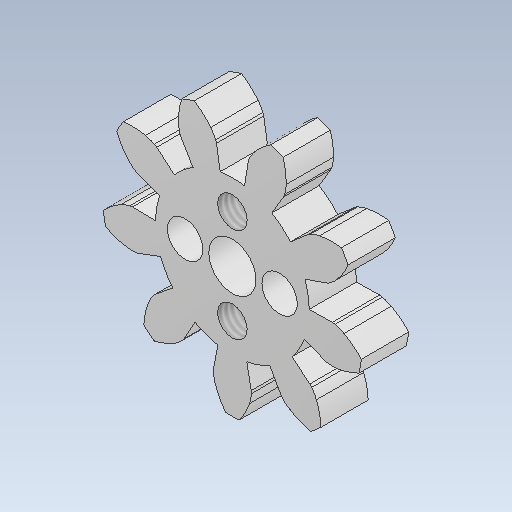
# Autodesk Inventor part: ｍ2歯数9ギアd3.99
Saved by Autodesk Inventor 2020.2 (Build 242310000, 310)
## iProperties
Created: 2020-03-11
Part Number: ｍ2歯数9ギアd3.99
Material: アルミニウム 2014-T4
Document SubType Name: Modeling
Designer: aoyam
Density: 2.8 g/cm^3
Appearance: サテン
Mass: 2.2827 g
Surface Area: 10.6305 cm^2
Volume: 0.815251 cm^3
Author: aoyam
Autodesk Inventor part; units mm, degrees
ref_plane "YZ Plane" through (0, 0, 0) normal (1, 0, 0) x (0, 1, 0)
ref_plane "XZ Plane" through (0, 0, 0) normal (0, 1, 0) x (-1, 0, 0)
ref_plane "XY Plane" through (0, 0, 0) normal (0, 0, 1) x (1, 0, 0)
sketch "スケッチ1" plane through (0, 0, 0) normal (0, 0, 1) x (1, 0, 0)
  arc A0 (8.759, 12.6536) -> (8.6861, 12.4312) centre (9.7767, 12.197) ccw
  arc A1 (9.1794, 13.3512) -> (8.759, 12.6536) centre (11.6212, 11.4041) ccw
  arc A2 (10.5668, 14.5981) -> (9.1794, 13.3512) centre (13.5776, 9.8526) ccw
  arc A3 (5.9975, 12.4312) -> (5.9246, 12.6536) centre (4.9069, 12.197) ccw
  arc A4 (5.9246, 12.6536) -> (5.5042, 13.3512) centre (3.0623, 11.4041) ccw
  arc A5 (5.5042, 13.3512) -> (4.1168, 14.5981) centre (1.106, 9.8526) ccw
  arc A6 (8.375, 10.4988) -> (6.3086, 10.4988) centre (7.3418, 4.0815) ccw
  arc A7 (4.1168, 14.5981) -> (3.0523, 14.2107) centre (7.3418, 4.0815) ccw
  line L0 (8.375, 10.4988) -> (8.6861, 12.4312)
  line L1 (6.3086, 10.4988) -> (5.9975, 12.4312)
  line L2 (2.4253, 8.3333) -> (0.9449, 9.6136)
  arc A8 (0.9449, 9.6136) -> (0.7461, 9.7372) centre (0.26, 8.7332) ccw
  arc A9 (0.7461, 9.7372) -> (-0.0244, 10.0013) centre (-0.6433, 6.9401) ccw
  arc A10 (-0.0244, 10.0013) -> (-1.8887, 10.0647) centre (-1.1447, 4.4942) ccw
  arc A11 (-1.8887, 10.0647) -> (-2.455, 9.0837) centre (7.3418, 4.0815) ccw
  arc A12 (2.9173, 11.5591) -> (3.0045, 11.3418) centre (3.9905, 11.8635) ccw
  arc A13 (4.0083, 9.6616) -> (2.4253, 8.3333) centre (7.3418, 4.0815) ccw
  line L3 (4.0083, 9.6616) -> (3.0045, 11.3418)
  arc A14 (2.791, 12.3637) -> (2.9173, 11.5591) centre (5.9132, 12.4417) ccw
  arc A15 (3.0523, 14.2107) -> (2.791, 12.3637) centre (8.409, 12.5107) ccw
  line L4 (0.8425, 4.1783) -> (-1.1145, 4.2075)
  arc A16 (-1.1145, 4.2075) -> (-1.3462, 4.1744) centre (-1.0733, 3.0928) ccw
  arc A17 (-1.3462, 4.1744) -> (-2.1062, 3.8815) centre (-0.6127, 1.1386) ccw
  arc A18 (-2.1062, 3.8815) -> (-3.5751, 2.7316) centre (0.5755, -1.0574) ccw
  arc A19 (-3.5751, 2.7316) -> (-3.3784, 1.6161) centre (7.3418, 4.0815) ccw
  arc A20 (-0.8541, 6.9657) -> (-0.6476, 6.8552) centre (-0.2276, 7.8886) ccw
  arc A21 (1.2013, 6.2133) -> (0.8425, 4.1783) centre (7.3418, 4.0815) ccw
  line L5 (1.2013, 6.2133) -> (-0.6476, 6.8552)
  arc A22 (-1.468, 7.5008) -> (-0.8541, 6.9657) centre (0.8736, 9.5675) ccw
  arc A23 (-2.455, 9.0837) -> (-1.468, 7.5008) centre (2.7411, 11.2246) ccw
  line L6 (2.3008, -0.022) -> (0.7829, -1.2576)
  arc A24 (0.7829, -1.2576) -> (0.6267, -1.4319) centre (1.531, -2.085) ccw
  arc A25 (0.6267, -1.4319) -> (0.2328, -2.1448) centre (3.14, -3.286) ccw
  arc A26 (0.2328, -2.1448) -> (-0.1534, -3.9698) centre (5.4617, -4.2045) ccw
  arc A27 (-0.1534, -3.9698) -> (0.7144, -4.6979) centre (7.3418, 4.0815) ccw
  arc A28 (-0.7905, 1.0227) -> (-0.5614, 1.0708) centre (-0.9039, 2.1324) ccw
  arc A29 (1.2676, 1.7675) -> (2.3008, -0.022) centre (7.3418, 4.0815) ccw
  line L7 (1.2676, 1.7675) -> (-0.5614, 1.0708)
  arc A30 (-1.6048, 1.038) -> (-0.7905, 1.0227) centre (-1.1395, 4.1263) ccw
  arc A31 (-3.3784, 1.6161) -> (-1.6048, 1.038) centre (-0.7741, 6.5962) ccw
  line L8 (6.1178, -2.3023) -> (5.7492, -4.2245)
  arc A32 (5.7492, -4.2245) -> (5.7416, -4.4585) centre (6.8542, -4.3774) ccw
  arc A33 (5.7416, -4.4585) -> (5.8981, -5.2577) centre (8.8587, -4.2632) ccw
  arc A34 (5.8981, -5.2577) -> (6.7754, -6.9039) centre (11.2276, -3.4744) ccw
  arc A35 (6.7754, -6.9039) -> (7.9082, -6.9039) centre (7.3418, 4.0815) ccw
  arc A36 (3.0782, -3.489) -> (3.2228, -3.3049) centre (2.278, -2.7119) ccw
  arc A37 (4.176, -1.5955) -> (6.1178, -2.3023) centre (7.3418, 4.0815) ccw
  line L9 (4.176, -1.5955) -> (3.2228, -3.3049)
  arc A38 (2.4446, -4.0008) -> (3.0782, -3.489) centre (0.8159, -1.3359) ccw
  arc A39 (0.7144, -4.6979) -> (2.4446, -4.0008) centre (-0.4918, 0.7911) ccw
  line L10 (10.5075, -1.5955) -> (11.4608, -3.3049)
  arc A40 (11.4608, -3.3049) -> (11.6054, -3.489) centre (12.4055, -2.7119) ccw
  arc A41 (11.6054, -3.489) -> (12.239, -4.0008) centre (13.8676, -1.3359) ccw
  arc A42 (12.239, -4.0008) -> (13.9692, -4.6979) centre (15.1754, 0.7911) ccw
  arc A43 (13.9692, -4.6979) -> (14.8369, -3.9698) centre (7.3418, 4.0815) ccw
  arc A44 (8.9419, -4.4585) -> (8.9343, -4.2245) centre (7.8294, -4.3774) ccw
  arc A45 (8.5658, -2.3023) -> (10.5075, -1.5955) centre (7.3418, 4.0815) ccw
  line L11 (8.5658, -2.3023) -> (8.9343, -4.2245)
  arc A46 (8.7855, -5.2577) -> (8.9419, -4.4585) centre (5.8249, -4.2632) ccw
  arc A47 (7.9082, -6.9039) -> (8.7855, -5.2577) centre (3.4559, -3.4744) ccw
  line L12 (13.416, 1.7675) -> (15.245, 1.0708)
  arc A48 (15.245, 1.0708) -> (15.4741, 1.0227) centre (15.5875, 2.1324) ccw
  arc A49 (15.4741, 1.0227) -> (16.2884, 1.038) centre (15.8231, 4.1263) ccw
  arc A50 (16.2884, 1.038) -> (18.062, 1.6161) centre (15.4577, 6.5962) ccw
  arc A51 (18.062, 1.6161) -> (18.2587, 2.7316) centre (7.3418, 4.0815) ccw
  arc A52 (14.0569, -1.4319) -> (13.9007, -1.2576) centre (13.1526, -2.085) ccw
  arc A53 (12.3828, -0.022) -> (13.416, 1.7675) centre (7.3418, 4.0815) ccw
  line L13 (12.3828, -0.022) -> (13.9007, -1.2576)
  arc A54 (14.4508, -2.1448) -> (14.0569, -1.4319) centre (11.5436, -3.286) ccw
  arc A55 (14.8369, -3.9698) -> (14.4508, -2.1448) centre (9.2219, -4.2045) ccw
  line L14 (13.4822, 6.2133) -> (15.3312, 6.8552)
  arc A56 (15.3312, 6.8552) -> (15.5376, 6.9657) centre (14.9112, 7.8886) ccw
  arc A57 (15.5376, 6.9657) -> (16.1516, 7.5008) centre (13.81, 9.5675) ccw
  arc A58 (16.1516, 7.5008) -> (17.1386, 9.0837) centre (11.9425, 11.2246) ccw
  arc A59 (17.1386, 9.0837) -> (16.5722, 10.0647) centre (7.3418, 4.0815) ccw
  arc A60 (16.0298, 4.1744) -> (15.7981, 4.2075) centre (15.7569, 3.0928) ccw
  arc A61 (13.8411, 4.1783) -> (13.4822, 6.2133) centre (7.3418, 4.0815) ccw
  line L15 (13.8411, 4.1783) -> (15.7981, 4.2075)
  arc A62 (16.7898, 3.8815) -> (16.0298, 4.1744) centre (15.2963, 1.1386) ccw
  arc A63 (18.2587, 2.7316) -> (16.7898, 3.8815) centre (14.1081, -1.0574) ccw
  line L16 (10.6753, 9.6616) -> (11.6791, 11.3418)
  arc A64 (11.6791, 11.3418) -> (11.7663, 11.5591) centre (10.6931, 11.8635) ccw
  arc A65 (11.7663, 11.5591) -> (11.8926, 12.3637) centre (8.7704, 12.4417) ccw
  arc A66 (11.8926, 12.3637) -> (11.6312, 14.2107) centre (6.2746, 12.5107) ccw
  arc A67 (11.6312, 14.2107) -> (10.5668, 14.5981) centre (7.3418, 4.0815) ccw
  arc A68 (13.9375, 9.7372) -> (13.7387, 9.6136) centre (14.4236, 8.7332) ccw
  arc A69 (12.2583, 8.3333) -> (10.6753, 9.6616) centre (7.3418, 4.0815) ccw
  line L17 (12.2583, 8.3333) -> (13.7387, 9.6136)
  arc A70 (14.7079, 10.0013) -> (13.9375, 9.7372) centre (15.3269, 6.9401) ccw
  arc A71 (16.5722, 10.0647) -> (14.7079, 10.0013) centre (15.8283, 4.4942) ccw
  circle A72 centre (7.3418, 4.0815) radius 1.995
  point P0 (0, 0)
  point P1 (6.3086, 10.4988)
  point P2 (5.9975, 12.4312)
  point P3 (5.9246, 12.6536)
  point P4 (5.5094, 13.3447)
  point P5 (4.1168, 14.5981)
  point P6 (3.0523, 14.2107)
  point P7 (2.7912, 12.3553)
  point P8 (2.9173, 11.5591)
  point P9 (3.0045, 11.3418)
  point P10 (4.0083, 9.6616)
  point P11 (2.4253, 8.3333)
  point P12 (0.9449, 9.6136)
  point P13 (0.7461, 9.7372)
  point P14 (-0.0162, 9.9996)
  point P15 (-1.8887, 10.0647)
  point P16 (-2.455, 9.0837)
  point P17 (-1.4625, 7.4946)
  point P18 (-0.8541, 6.9657)
  point P19 (-0.6476, 6.8552)
  point P20 (1.2013, 6.2133)
  point P21 (0.8425, 4.1783)
  point P22 (-1.1145, 4.2075)
  point P23 (-1.3462, 4.1744)
  point P24 (-2.0989, 3.8854)
  point P25 (-3.5751, 2.7316)
  point P26 (-3.3784, 1.6161)
  point P27 (-1.5966, 1.0368)
  point P28 (-0.7905, 1.0227)
  point P29 (-0.5614, 1.0708)
  point P30 (2.3008, -0.022)
  point P31 (0.7829, -1.2576)
  point P32 (0.6267, -1.4319)
  point P33 (0.2358, -2.137)
  point P34 (-0.1534, -3.9698)
  point P35 (0.7144, -4.6979)
  point P36 (2.4517, -3.9964)
  point P37 (3.0782, -3.489)
  point P38 (3.2228, -3.3049)
  point P39 (6.1178, -2.3023)
  point P40 (5.7492, -4.2245)
  point P41 (5.7416, -4.4585)
  point P42 (5.8955, -5.2498)
  point P43 (6.7754, -6.9039)
  point P44 (7.9082, -6.9039)
  point P45 (8.7881, -5.2498)
  point P46 (8.9419, -4.4585)
  point P47 (8.9343, -4.2245)
  point P48 (8.5658, -2.3023)
  point P49 (11.6054, -3.489)
  point P50 (12.2319, -3.9964)
  point P51 (13.9692, -4.6979)
  point P52 (14.8369, -3.9698)
  point P53 (14.4478, -2.137)
  point P54 (14.0569, -1.4319)
  point P55 (13.9007, -1.2576)
  point P56 (12.3828, -0.022)
  point P57 (13.416, 1.7675)
  point P58 (15.4741, 1.0227)
  point P59 (16.2802, 1.0368)
  point P60 (18.062, 1.6161)
  point P61 (18.2587, 2.7316)
  point P62 (16.7825, 3.8854)
  point P63 (16.0298, 4.1744)
  point P64 (15.7981, 4.2075)
  point P65 (13.8411, 4.1783)
  point P66 (15.5376, 6.9657)
  point P67 (16.1461, 7.4946)
  point P68 (17.1386, 9.0837)
  point P69 (16.5722, 10.0647)
  point P70 (14.6998, 9.9996)
  point P71 (13.9375, 9.7372)
  point P72 (11.7663, 11.5591)
  point P73 (11.8924, 12.3553)
  point P74 (10.5668, 14.5981)
  point P75 (9.1742, 13.3447)
  point P76 (8.759, 12.6536)
  dimension "d2" = 360
  dimension "d4" = 3.99
  constraints: 144 point on circle, 73 centre point, 36 end point, 3 coincident, 341 other
  measures "d4" diameter of A72
extrude "押し出し1" add sketch "スケッチ1" along normal blind 4
sketch "スケッチ4" plane through (0, 0, 4) normal (0, 0, 1) x (1, 0, 0)
  arc A0 (5.9975, 12.4312) -> (5.9246, 12.6536) centre (4.9069, 12.197) ccw projected
  arc A1 (5.9246, 12.6536) -> (5.5094, 13.3447) centre (3.0623, 11.4041) ccw projected
  arc A2 (5.5094, 13.3447) -> (4.1168, 14.5981) centre (1.106, 9.8526) ccw projected
  arc A3 (4.1168, 14.5981) -> (3.0523, 14.2107) centre (7.3418, 4.0815) ccw projected
  arc A4 (3.0523, 14.2107) -> (2.791, 12.3637) centre (8.409, 12.5107) ccw projected
  arc A5 (2.791, 12.3637) -> (2.9173, 11.5591) centre (5.9132, 12.4417) ccw projected
  arc A6 (2.9173, 11.5591) -> (3.0045, 11.3418) centre (3.9905, 11.8635) ccw projected
  line L0 (3.0045, 11.3418) -> (4.0083, 9.6616) projected
  arc A7 (4.0083, 9.6616) -> (2.4253, 8.3333) centre (7.3418, 4.0815) ccw projected
  line L1 (2.4253, 8.3333) -> (0.9449, 9.6136) projected
  arc A8 (0.9449, 9.6136) -> (0.7461, 9.7372) centre (0.26, 8.7332) ccw projected
  arc A9 (0.7461, 9.7372) -> (-0.0162, 9.9996) centre (-0.6433, 6.9401) ccw projected
  arc A10 (-0.0162, 9.9996) -> (-1.8887, 10.0647) centre (-1.1447, 4.4942) ccw projected
  arc A11 (-1.8887, 10.0647) -> (-2.455, 9.0837) centre (7.3418, 4.0815) ccw projected
  arc A12 (-2.455, 9.0837) -> (-1.468, 7.5008) centre (2.7411, 11.2246) ccw projected
  arc A13 (-1.468, 7.5008) -> (-0.8541, 6.9657) centre (0.8736, 9.5675) ccw projected
  arc A14 (-0.8541, 6.9657) -> (-0.6476, 6.8552) centre (-0.2276, 7.8886) ccw projected
  line L2 (-0.6476, 6.8552) -> (1.2013, 6.2133) projected
  arc A15 (1.2013, 6.2133) -> (0.8425, 4.1783) centre (7.3418, 4.0815) ccw projected
  line L3 (0.8425, 4.1783) -> (-1.1145, 4.2075) projected
  arc A16 (-1.1145, 4.2075) -> (-1.3462, 4.1744) centre (-1.0733, 3.0928) ccw projected
  arc A17 (-1.3462, 4.1744) -> (-2.0989, 3.8854) centre (-0.6127, 1.1386) ccw projected
  arc A18 (-2.0989, 3.8854) -> (-3.5751, 2.7316) centre (0.5755, -1.0574) ccw projected
  arc A19 (-3.5751, 2.7316) -> (-3.3784, 1.6161) centre (7.3418, 4.0815) ccw projected
  arc A20 (-3.3784, 1.6161) -> (-1.6048, 1.038) centre (-0.7741, 6.5962) ccw projected
  arc A21 (-1.6048, 1.038) -> (-0.7905, 1.0227) centre (-1.1395, 4.1263) ccw projected
  arc A22 (-0.7905, 1.0227) -> (-0.5614, 1.0708) centre (-0.9039, 2.1324) ccw projected
  line L4 (-0.5614, 1.0708) -> (1.2676, 1.7675) projected
  arc A23 (1.2676, 1.7675) -> (2.3008, -0.022) centre (7.3418, 4.0815) ccw projected
  line L5 (2.3008, -0.022) -> (0.7829, -1.2576) projected
  arc A24 (0.7829, -1.2576) -> (0.6267, -1.4319) centre (1.531, -2.085) ccw projected
  arc A25 (0.6267, -1.4319) -> (0.2358, -2.137) centre (3.14, -3.286) ccw projected
  arc A26 (0.2358, -2.137) -> (-0.1534, -3.9698) centre (5.4617, -4.2045) ccw projected
  arc A27 (-0.1534, -3.9698) -> (0.7144, -4.6979) centre (7.3418, 4.0815) ccw projected
  arc A28 (0.7144, -4.6979) -> (2.4446, -4.0008) centre (-0.4918, 0.7911) ccw projected
  arc A29 (2.4446, -4.0008) -> (3.0782, -3.489) centre (0.8159, -1.3359) ccw projected
  arc A30 (3.0782, -3.489) -> (3.2228, -3.3049) centre (2.278, -2.7119) ccw projected
  line L6 (3.2228, -3.3049) -> (4.176, -1.5955) projected
  arc A31 (4.176, -1.5955) -> (6.1178, -2.3023) centre (7.3418, 4.0815) ccw projected
  line L7 (6.1178, -2.3023) -> (5.7492, -4.2245) projected
  arc A32 (5.7492, -4.2245) -> (5.7416, -4.4585) centre (6.8542, -4.3774) ccw projected
  arc A33 (5.7416, -4.4585) -> (5.8955, -5.2498) centre (8.8587, -4.2632) ccw projected
  arc A34 (5.8955, -5.2498) -> (6.7754, -6.9039) centre (11.2276, -3.4744) ccw projected
  arc A35 (6.7754, -6.9039) -> (7.9082, -6.9039) centre (7.3418, 4.0815) ccw projected
  arc A36 (7.9082, -6.9039) -> (8.7855, -5.2577) centre (3.4559, -3.4744) ccw projected
  arc A37 (8.7855, -5.2577) -> (8.9419, -4.4585) centre (5.8249, -4.2632) ccw projected
  arc A38 (8.9419, -4.4585) -> (8.9343, -4.2245) centre (7.8294, -4.3774) ccw projected
  line L8 (8.9343, -4.2245) -> (8.5658, -2.3023) projected
  arc A39 (8.5658, -2.3023) -> (10.5075, -1.5955) centre (7.3418, 4.0815) ccw projected
  line L9 (10.5075, -1.5955) -> (11.4608, -3.3049) projected
  arc A40 (11.4608, -3.3049) -> (11.6054, -3.489) centre (12.4055, -2.7119) ccw projected
  arc A41 (11.6054, -3.489) -> (12.2319, -3.9964) centre (13.8676, -1.3359) ccw projected
  arc A42 (12.2319, -3.9964) -> (13.9692, -4.6979) centre (15.1754, 0.7911) ccw projected
  arc A43 (13.9692, -4.6979) -> (14.8369, -3.9698) centre (7.3418, 4.0815) ccw projected
  arc A44 (14.8369, -3.9698) -> (14.4508, -2.1448) centre (9.2219, -4.2045) ccw projected
  arc A45 (14.4508, -2.1448) -> (14.0569, -1.4319) centre (11.5436, -3.286) ccw projected
  arc A46 (14.0569, -1.4319) -> (13.9007, -1.2576) centre (13.1526, -2.085) ccw projected
  line L10 (13.9007, -1.2576) -> (12.3828, -0.022) projected
  arc A47 (12.3828, -0.022) -> (13.416, 1.7675) centre (7.3418, 4.0815) ccw projected
  line L11 (13.416, 1.7675) -> (15.245, 1.0708) projected
  arc A48 (15.245, 1.0708) -> (15.4741, 1.0227) centre (15.5875, 2.1324) ccw projected
  arc A49 (15.4741, 1.0227) -> (16.2802, 1.0368) centre (15.8231, 4.1263) ccw projected
  arc A50 (16.2802, 1.0368) -> (18.062, 1.6161) centre (15.4577, 6.5962) ccw projected
  arc A51 (18.062, 1.6161) -> (18.2587, 2.7316) centre (7.3418, 4.0815) ccw projected
  arc A52 (18.2587, 2.7316) -> (16.7898, 3.8815) centre (14.1081, -1.0574) ccw projected
  arc A53 (16.7898, 3.8815) -> (16.0298, 4.1744) centre (15.2963, 1.1386) ccw projected
  arc A54 (16.0298, 4.1744) -> (15.7981, 4.2075) centre (15.7569, 3.0928) ccw projected
  line L12 (15.7981, 4.2075) -> (13.8411, 4.1783) projected
  arc A55 (13.8411, 4.1783) -> (13.4822, 6.2133) centre (7.3418, 4.0815) ccw projected
  line L13 (13.4822, 6.2133) -> (15.3312, 6.8552) projected
  arc A56 (15.3312, 6.8552) -> (15.5376, 6.9657) centre (14.9112, 7.8886) ccw projected
  arc A57 (15.5376, 6.9657) -> (16.1461, 7.4946) centre (13.81, 9.5675) ccw projected
  arc A58 (16.1461, 7.4946) -> (17.1386, 9.0837) centre (11.9425, 11.2246) ccw projected
  arc A59 (17.1386, 9.0837) -> (16.5722, 10.0647) centre (7.3418, 4.0815) ccw projected
  arc A60 (16.5722, 10.0647) -> (14.7079, 10.0013) centre (15.8283, 4.4942) ccw projected
  arc A61 (14.7079, 10.0013) -> (13.9375, 9.7372) centre (15.3269, 6.9401) ccw projected
  arc A62 (13.9375, 9.7372) -> (13.7387, 9.6136) centre (14.4236, 8.7332) ccw projected
  line L14 (13.7387, 9.6136) -> (12.2583, 8.3333) projected
  arc A63 (12.2583, 8.3333) -> (10.6753, 9.6616) centre (7.3418, 4.0815) ccw projected
  line L15 (10.6753, 9.6616) -> (11.6791, 11.3418) projected
  arc A64 (11.6791, 11.3418) -> (11.7663, 11.5591) centre (10.6931, 11.8635) ccw projected
  arc A65 (11.7663, 11.5591) -> (11.8924, 12.3553) centre (8.7704, 12.4417) ccw projected
  arc A66 (11.8924, 12.3553) -> (11.6312, 14.2107) centre (6.2746, 12.5107) ccw projected
  arc A67 (11.6312, 14.2107) -> (10.5668, 14.5981) centre (7.3418, 4.0815) ccw projected
  arc A68 (10.5668, 14.5981) -> (9.1794, 13.3512) centre (13.5776, 9.8526) ccw projected
  arc A69 (9.1794, 13.3512) -> (8.759, 12.6536) centre (11.6212, 11.4041) ccw projected
  arc A70 (8.759, 12.6536) -> (8.6861, 12.4312) centre (9.7767, 12.197) ccw projected
  line L16 (8.6861, 12.4312) -> (8.375, 10.4988) projected
  arc A71 (8.375, 10.4988) -> (6.3086, 10.4988) centre (7.3418, 4.0815) ccw projected
  line L17 (6.3086, 10.4988) -> (5.9975, 12.4312) projected
  circle A72 centre (7.3418, 4.0815) radius 1.995 projected
  circle A73 centre (7.3418, 8.0815) radius 1.25
  circle A74 centre (7.3418, 0.0815) radius 1.25
  circle A75 centre (3.3418, 4.0815) radius 1.5
  line L18 (7.3418, 4.0815) -> (7.3418, 8.0815)
  line L19 (3.3418, 4.0815) -> (7.3418, 4.0815)
  circle A76 centre (11.3418, 4.0815) radius 1.5
  point P0 (0, 0)
  dimension "d38" = 2.5
  dimension "d42" = 360
  dimension "d57" = 3
  dimension "d58" = 4
  dimension "d59" = 4
  dimension "d62" = 360
  constraints: 4 centre point, 4 end point, 2 coincident, 1 horizontal, 1 vertical, 10 other
  measures "d38" diameter of A73
  measures "d57" diameter of A75
  measures "d58" distance of L18.start L18.end
  measures "d59" distance of L19.start L19.end
extrude "押し出し4" cut sketch "スケッチ4" against normal blind 4 contours A75 | A73 | A74 | A76
thread "ねじ9" size "M3x0.5" class "6H" standard "ANSI Metric M Profile" length 44.8
thread "ねじ10" size "M3x0.5" class "6H" standard "ANSI Metric M Profile" length 44.8
